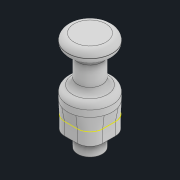
# Autodesk Inventor part: guia
Saved by Autodesk Inventor 2021 (Build 250183000, 183)
## iProperties
Created: 2021-12-18
Part Number: guia
Material: Generic
Document SubType Name: Modeling
Designer: Juan M. Casillas
Density: 1 g/cm^3
Appearance: Default
Author: Juan M. Casillas
Autodesk Inventor part; units mm, degrees
ref_plane "YZ Plane" through (0, 0, 0) normal (1, 0, 0) x (0, 1, 0)
ref_plane "XZ Plane" through (0, 0, 0) normal (0, 1, 0) x (-1, 0, 0)
ref_plane "XY Plane" through (0, 0, 0) normal (0, 0, 1) x (1, 0, 0)
sketch "Sketch1" plane through (0, 0, 0) normal (0, 1, 0) x (-1, 0, 0)
  circle A0 centre (0, 0) radius 1.925
  dimension "d0" = 3.85
  constraints: 1 centre point, 1 coincident
  measures "d0" diameter of A0
extrude "Extrusion1" add sketch "Sketch1" along normal blind 2.5
sketch "Sketch2" plane through (0, 2.5, 0) normal (0, 1, 0) x (1, 0, 0)
  line L0 (-1, -3) -> (1, -3)
  line L1 (3, -1) -> (3, 1)
  line L2 (1, 3) -> (-1, 3)
  line L3 (-3, 1) -> (-3, -1)
  line L4 (-3, -3) -> (3, 3) construction
  line L5 (3, -3) -> (-3, 3) construction
  arc A0 (-3, -1) -> (-1, -3) centre (-1, -1) ccw
  arc A1 (-1, 3) -> (-3, 1) centre (-1, 1) ccw
  arc A2 (3, 1) -> (1, 3) centre (1, 1) ccw
  arc A3 (1, -3) -> (3, -1) centre (1, -1) ccw
  point P0 (0, 0)
  dimension "d3" = 6
  dimension "d4" = 6
  dimension "d5" = 2
  constraints: 12 end point, 8 point on circle, 8 point on line, 8 tangent, 4 centre point, 3 equal radius, 2 midpoint, 2 parallel, 1 horizontal, 1 perpendicular
  measures "d3" distance of L5.end L4.end
  measures "d4" distance of L4.end L5.start
  measures "d5" radius of A0
extrude "Extrusion2" add sketch "Sketch2" along normal blind 2
sketch "Sketch3" plane through (0, 4.5, 0) normal (0, 1, 0) x (1, 0, 0)
  circle A0 centre (0, 0) radius 1.925 projected
extrude "Extrusion3" add sketch "Sketch3" along normal blind 2
sketch "Sketch5" plane through (0, 6.5, 0) normal (0, 1, 0) x (1, 0, 0)
  circle A0 centre (0, 0) radius 3.5
  dimension "d14" = 7
  constraints: 1 centre point, 1 coincident
  measures "d14" diameter of A0
extrude "Extrusion5" add sketch "Sketch5" along normal blind 2
sketch "Sketch6" plane through (0, 8.5, 0) normal (0, 1, 0) x (1, 0, 0)
  circle A0 centre (0, 0) radius 1.925 projected
extrude "Extrusion6" add sketch "Sketch6" along normal blind 5
sketch "Sketch7" plane through (0, 13.5, 0) normal (0, 1, 0) x (1, 0, 0)
  circle A0 centre (0, 0) radius 3.5 projected
extrude "Extrusion7" add sketch "Sketch7" along normal blind 2
sketch "Sketch8" plane through (0, 4.5, 0) normal (0, 1, 0) x (1, 0, 0)
  circle A0 centre (0, 0) radius 1.925 projected
  arc A1 (1, -3) -> (3, -1) centre (1, -1) ccw projected
  line L0 (3, -1) -> (3, 1) projected
  arc A2 (3, 1) -> (1, 3) centre (1, 1) ccw projected
  line L1 (1, 3) -> (-1, 3) projected
  arc A3 (-1, 3) -> (-3, 1) centre (-1, 1) ccw projected
  line L2 (-3, 1) -> (-3, -1) projected
  arc A4 (-3, -1) -> (-1, -3) centre (-1, -1) ccw projected
  line L3 (-1, -3) -> (1, -3) projected
loft "Loft1" add section 1 edges at (2.4142, 4.5, 2.4142) (3, 4.5, 0) (2.4142, 4.5, -2.4142) (0, 4.5, -3) (-2.4142, 4.5, -2.4142) (-3, 4.5, 0) (-2.4142, 4.5, 2.4142) (0, 4.5, 3) section 2 edges at (-3.5, 6.5, 0)
fillet "Fillet3" radius 1 5 edges at (-3.5, 8.5, 0) (-1.925, 8.5, 0) (-1.925, 13.5, 0) (-3.5, 13.5, 0) (-3.5, 15.5, 0)
body "Solid1"
